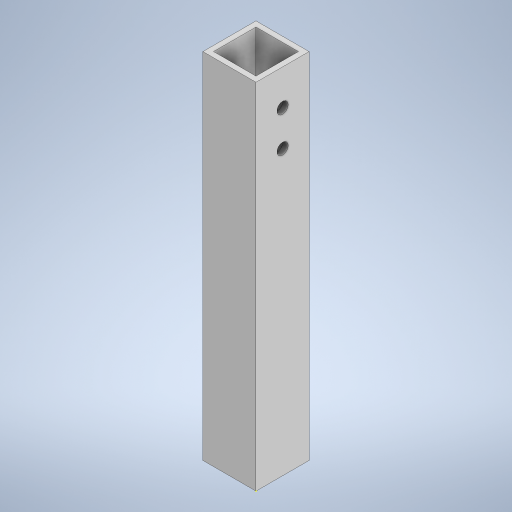
# Autodesk Inventor part: Part1
Saved by Autodesk Inventor 2023 (Build 270158000, 158)
## iProperties
Created: 2022-04-25
Part Number: Part1
Material: 一般
Document SubType Name: Modeling
Designer: yuta
Density: 1 g/cm^3
Appearance: 既定
Author: yuta
Autodesk Inventor part; units mm, degrees
ref_plane "YZ Plane" through (0, 0, 0) normal (1, 0, 0) x (0, 1, 0)
ref_plane "XZ Plane" through (0, 0, 0) normal (0, 1, 0) x (-1, 0, 0)
ref_plane "XY Plane" through (0, 0, 0) normal (0, 0, 1) x (1, 0, 0)
sketch "スケッチ1" plane through (0, 0, 0) normal (0, 1, 0) x (-1, 0, 0)
  line L0 (0, 0) -> (15, 0)
  line L1 (15, 0) -> (15, -15)
  line L2 (15, -15) -> (0, -15)
  line L3 (0, -15) -> (0, 0)
  dimension "d0" = 15
  dimension "d1" = 15
  constraints: 8 end point, 2 parallel, 1 horizontal, 1 perpendicular
  measures "d0" distance of L1.end L2.end
  measures "d1" distance of L0.end L1.end
extrude "押し出し1" add sketch "スケッチ1" along normal blind 100
sketch "スケッチ2" plane through (0, 100, 0) normal (0, 1, 0) x (1, 0, 0)
  line L0 (-13.5, 13.5) -> (-1.5, 13.5)
  line L1 (-1.5, 13.5) -> (-1.5, 1.5)
  line L2 (-1.5, 1.5) -> (-13.5, 1.5)
  line L3 (-13.5, 1.5) -> (-13.5, 13.5)
  line L4 (-15, 15) -> (-15, 0) projected
  line L5 (0, 15) -> (-15, 15) projected
  point P0 (0, 0)
  dimension "d4" = 12
  dimension "d5" = 12
  dimension "d6" = 1.5
  dimension "d7" = 1.5
  constraints: 8 end point, 2 parallel, 1 horizontal, 1 perpendicular
  measures "d4" distance of L1.end L2.end
  measures "d5" distance of L0.end L1.end
  measures "d6" distance between parallel lines of L4 L3
  measures "d7" distance between parallel lines of L5 L0
extrude "押し出し2" cut sketch "スケッチ2" against normal blind 100
sketch "スケッチ3" plane through (0, 0, 0) normal (1, 0, 0) x (0, 0, -1)
  point P0 (0, 0)
sketch "スケッチ4" plane through (0, 0, 0) normal (1, 0, 0) x (0, 0, -1)
  line L0 (0, 100) -> (15, 100) projected
  line L1 (0, 0) -> (0, 100) projected
  point P0 (7.5, 90)
  point P1 (7.5, 80)
  dimension "d10" = 10
  dimension "d11" = 7.5
  dimension "d12" = 10
  dimension "d13" = 7.5
  measures "d10" distance from line of L0 point (7.5, 90)
  measures "d11" distance from line of L1 point (7.5, 90)
  measures "d12" distance of point (7.5, 80) point (7.5, 90)
  measures "d13" distance from line of L1 point (7.5, 80)
hole "穴1" at (0, 90, -7.5) at (0, 80, -7.5) direction (-1, 0, 0) diameter 3.2 end through all
